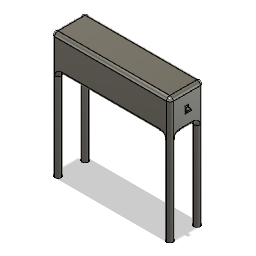
cat v1 (Autodesk Fusion 360 design; units mm, degrees)
Autodesk Fusion 360 part; units mm, degrees
sketch "Sketch1" plane through (0, 0, 0) normal (0, 1, 0) x (1, 0, 0)
  line L0 (0, 0) -> (350, 0)
  line L1 (350, 0) -> (350, 100)
  line L2 (350, 100) -> (0, 100)
  line L3 (0, 100) -> (0, 0)
  line L4 (0, 0) -> (20, 0)
  line L5 (20, 0) -> (20, 20)
  line L6 (20, 20) -> (0, 20)
  line L7 (0, 20) -> (0, 0)
  line L8 (0, 100) -> (20, 100)
  line L9 (20, 100) -> (20, 80)
  line L10 (20, 80) -> (0, 80)
  line L11 (0, 80) -> (0, 100)
  line L12 (350, 100) -> (330, 100)
  line L13 (330, 100) -> (330, 80)
  line L14 (330, 80) -> (350, 80)
  line L15 (350, 80) -> (350, 100)
  line L16 (350, 0) -> (330, 0)
  line L17 (330, 0) -> (330, 20)
  line L18 (330, 20) -> (350, 20)
  line L19 (350, 20) -> (350, 0)
  dimension "d1" = 350
  dimension "d2" = 100
  dimension "d3" = 20
  dimension "d4" = 20
  dimension "d5" = 20
  dimension "d6" = 20
  dimension "d7" = 20
  dimension "d8" = 20
  dimension "d9" = 20
  dimension "d10" = 20
  constraint horizontal L0
  constraint vertical L1
  constraint horizontal L2
  constraint vertical L3
  constraint coincident L0.start L3.end
  constraint horizontal L4
  constraint vertical L5
  constraint horizontal L6
  constraint vertical L7
  constraint horizontal L8
  constraint vertical L9
  constraint horizontal L10
  constraint vertical L11
  constraint horizontal L12
  constraint vertical L13
  constraint horizontal L14
  constraint vertical L15
  constraint horizontal L16
  constraint vertical L17
  constraint horizontal L18
  constraint vertical L19
  measures "d1" distance of L0.start L0.end
  measures "d2" distance of L0.start L2.end
  measures "d3" distance of L0.start L4.end
  measures "d4" distance of L0.start L6.end
  measures "d5" distance of L2.end L8.end
  measures "d6" distance of L2.end L10.end
  measures "d7" distance of L1.end L12.end
  measures "d8" distance of L1.end L14.end
  measures "d9" distance of L0.end L16.end
  measures "d10" distance of L0.end L18.end
extrude "Extrude1" add sketch "Sketch1" along normal blind 100 makes body 1
sketch "Sketch2" plane through (0, 0, 0) normal (0, -1, 0) x (1, 0, 0)
  line L0 (350, -100) -> (350, 0)
  line L1 (350, 0) -> (0, 0)
  line L2 (0, 0) -> (0, -100)
  line L3 (0, -100) -> (350, -100)
  line L4 (350, -100) -> (330, -100)
  line L5 (330, -100) -> (330, -80)
  line L6 (330, -80) -> (350, -80)
  line L7 (350, -80) -> (350, -100)
  line L8 (350, 0) -> (330, 0)
  line L9 (330, 0) -> (330, -20)
  line L10 (330, -20) -> (350, -20)
  line L11 (350, -20) -> (350, 0)
  line L12 (0, 0) -> (20, 0)
  line L13 (20, 0) -> (20, -20)
  line L14 (20, -20) -> (0, -20)
  line L15 (0, -20) -> (0, 0)
  line L16 (0, -100) -> (20, -100)
  line L17 (20, -100) -> (20, -80)
  line L18 (20, -80) -> (0, -80)
  line L19 (0, -80) -> (0, -100)
  dimension "d13" = 20
  dimension "d14" = 20
  dimension "d15" = 20
  dimension "d16" = 20
  dimension "d17" = 20
  dimension "d18" = 20
  dimension "d19" = 20
  dimension "d20" = 20
  constraint horizontal L4
  constraint vertical L5
  constraint horizontal L6
  constraint vertical L7
  constraint coincident L0.start L3.end
  constraint horizontal L8
  constraint vertical L9
  constraint horizontal L10
  constraint vertical L11
  constraint coincident L0.end L1.start
  constraint horizontal L12
  constraint vertical L13
  constraint horizontal L14
  constraint vertical L15
  constraint coincident L1.end L2.start
  constraint horizontal L16
  constraint vertical L17
  constraint horizontal L18
  constraint vertical L19
  constraint coincident L2.end L3.start
  measures "d13" distance of L0.start L4.end
  measures "d14" distance of L0.start L6.end
  measures "d15" distance of L0.end L8.end
  measures "d16" distance of L0.end L10.end
  measures "d17" distance of L1.end L12.end
  measures "d18" distance of L1.end L14.end
  measures "d19" distance of L2.end L16.end
  measures "d20" distance of L2.end L18.end
extrude "Extrude2" add sketch "Sketch2" along normal blind 300 contours L0 L3 L4 L5 L6 L7 | L0 L1 L8 L9 L10 L11 | L2 L3 L16 L17 L18 L19 | L1 L2 L12 L13 L14 L15 bodies 1
move_body "Move1" bodies 1 to x (1, 0, 0) y (0, 1, 0) z (0, 0, 1) at (0, 300, 0)
fillet "Fillet1" radius 9.9 40 edges at (350, 200, 0) (20, 150, 0) (20, 300, -10) (175, 300, 0) (330, 300, -90) (330, 0, -90) (340, 300, -80) (0, 0, -10) (0, 200, 0) (350, 400, -50) (350, 300, -50) (330, 0, -10) (330, 300, -10) (340, 300, -20) (350, 0, -90) (350, 0, -10) (330, 150, 0) (0, 150, -80) (350, 150, -20) (0, 300, -50) (350, 150, -80) (0, 150, -20) (175, 400, -100) (175, 400, 0) (330, 150, -100) (0, 200, -100) (330, 150, -20) (0, 400, -50) (330, 150, -80) (0, 0, -90) (350, 200, -100) (20, 150, -80) (20, 0, -90) (20, 0, -10) (20, 150, -20) (10, 300, -20) (10, 300, -80) (20, 300, -90) (175, 300, -100) (20, 150, -100) on bodies 1
sketch "Sketch3" plane through (0, 0, 0) normal (0, 1, 0) x (1, 0, 0)
  line L0 (-15, 5) -> (385, 5)
  line L1 (385, 5) -> (385, 15)
  line L2 (385, 15) -> (-15, 15)
  line L3 (-15, 15) -> (-15, 5)
  dimension "d25" = 400
  dimension "d26" = 10
  constraint horizontal L0
  constraint vertical L1
  constraint horizontal L2
  constraint vertical L3
  measures "d25" distance of L0.start L0.end
  measures "d26" distance of L0.start L2.end
extrude "Extrude3" cut sketch "Sketch3" along normal blind 30 bodies 1
sketch "Sketch4" plane through (0, 0, 0) normal (0, 1, 0) x (1, 0, 0)
  line L0 (-15, 95) -> (385, 95)
  line L1 (385, 95) -> (385, 85)
  line L2 (385, 85) -> (-15, 85)
  line L3 (-15, 85) -> (-15, 95)
  dimension "d29" = 400
  dimension "d30" = 10
  constraint horizontal L0
  constraint vertical L1
  constraint horizontal L2
  constraint vertical L3
  measures "d29" distance of L0.start L0.end
  measures "d30" distance of L0.start L2.end
extrude "Extrude4" cut sketch "Sketch4" along normal blind 30 bodies 1
sketch "Sketch5" plane through (0, 0, 0) normal (-1, 0, 0) x (0, 0, 1)
  line L0 (-90.1, 30) -> (-89.9, 30)
  line L1 (-89.9, 30) -> (-89.9, 290.1)
  arc A0 (-70.1, 309.9) -> (-89.9, 290.1) centre (-70.1, 290.1) ccw
  line L2 (-70.1, 309.9) -> (-29.9, 309.9)
  arc A1 (-10.1, 290.1) -> (-29.9, 309.9) centre (-29.9, 290.1) ccw
  line L3 (-10.1, 290.1) -> (-10.1, 30)
  line L4 (-10.1, 30) -> (-9.9, 30)
  line L5 (-9.9, 30) -> (-9.9, 390.1)
  line L6 (-9.9, 390.1) -> (-90.1, 390.1)
  line L7 (-90.1, 390.1) -> (-90.1, 30)
  circle A2 centre (-50, 350) radius 25
  line L8 (-70.1, 364.8657) -> (-85, 360)
  line L9 (-85, 360) -> (-75, 350)
  line L10 (-29.9, 364.8657) -> (-15, 360)
  line L11 (-15, 360) -> (-25, 350)
  line L12 (-45, 345) -> (-40, 350)
  line L13 (-40, 350) -> (-30, 350)
  line L14 (-30, 350) -> (-35, 345)
  line L15 (-35, 345) -> (-45, 345)
  line L16 (-55, 345) -> (-60, 350)
  line L17 (-60, 350) -> (-70, 350)
  line L18 (-70, 350) -> (-65, 345)
  line L19 (-65, 345) -> (-55, 345)
  line L20 (-48, 342) -> (-52, 342)
  line L21 (-52, 342) -> (-50, 340)
  line L22 (-50, 340) -> (-48, 342)
  line L23 (-50, 337) -> (-47, 335)
  line L24 (-47, 335) -> (-45, 336)
  line L25 (-45, 336) -> (-45, 335)
  line L26 (-45, 335) -> (-47, 334)
  line L27 (-47, 334) -> (-50, 336)
  line L28 (-50, 336) -> (-53, 334)
  line L29 (-53, 334) -> (-55, 335)
  line L30 (-55, 335) -> (-55, 336)
  line L31 (-55, 336) -> (-53, 335)
  line L32 (-53, 335) -> (-50, 337)
  dimension "d33" = 50
  constraint coincident A2 L8.start
  constraint coincident A2 L9.end
  constraint coincident A2 L10.start
  constraint coincident A2 L11.end
  constraint parallel L11 L12
  constraint horizontal L13
  constraint parallel L12 L14
  constraint parallel L13 L15
  constraint perpendicular L12 L16
  constraint parallel L15 L17
  constraint parallel L16 L18
  constraint parallel L17 L19
  constraint horizontal L20
  constraint perpendicular L21 L22
  constraint vertical L25
  constraint parallel L24 L26
  constraint vertical L30
  constraint parallel L29 L31
  measures "d33" diameter of A2
extrude "Extrude5" add sketch "Sketch5" along normal blind 5 contours A2 | A2 L10 L11 | A2 L8 L9 bodies 1
sketch "Sketch6" plane through (350, 0, 0) normal (1, 0, 0) x (0, 0, -1)
  line L0 (89.9, 30) -> (90.1, 30)
  line L1 (90.1, 30) -> (90.1, 390.1)
  line L2 (90.1, 390.1) -> (9.9, 390.1)
  line L3 (9.9, 390.1) -> (9.9, 30)
  line L4 (9.9, 30) -> (10.1, 30)
  line L5 (10.1, 30) -> (10.1, 290.1)
  arc A0 (29.9, 309.9) -> (10.1, 290.1) centre (29.9, 290.1) ccw
  line L6 (29.9, 309.9) -> (70.1, 309.9)
  arc A1 (89.9, 290.1) -> (70.1, 309.9) centre (70.1, 290.1) ccw
  line L7 (89.9, 290.1) -> (89.9, 30)
  line L8 (55, 360) -> (45, 360)
  line L9 (45, 360) -> (45, 340)
  line L10 (45, 340) -> (55, 340)
  line L11 (55, 340) -> (55, 360)
  constraint horizontal L8
  constraint vertical L9
  constraint horizontal L10
  constraint vertical L11
extrude "Extrude6" cut sketch "Sketch6" against normal blind 2 contours L8 L9 L10 L11 bodies 1
sketch "Sketch7" plane through (348, 0, 0) normal (1, 0, 0) x (0, 0, -1)
  line L0 (55, 340) -> (55, 360)
  line L1 (55, 360) -> (45, 360)
  line L2 (45, 360) -> (45, 340)
  line L3 (45, 340) -> (55, 340)
  line L4 (55, 352.0722) -> (45, 352.0722)
  line L5 (45, 352.0722) -> (45, 348.0722)
  line L6 (45, 348.0722) -> (55, 348.0722)
  line L7 (55, 348.0722) -> (55, 352.0722)
  dimension "d38" = 10
  dimension "d39" = 4
  constraint horizontal L4
  constraint vertical L5
  constraint horizontal L6
  constraint vertical L7
  constraint coincident L0 L4.start
  measures "d38" distance of L4.start L4.end
  measures "d39" distance of L4.start L6.end
extrude "Extrude7" add sketch "Sketch7" along normal blind 10 separate body contours L0 L2 L4 L5 L6 L7 makes body 2
extrude "Extrude8" cut 1 faces at (342.9008, 21.6667, -85) along direction (0, 0, -1) blind 45 on bodies 1 bodies 1
extrude "Extrude9" cut 1 faces at (12.9008, 21.6667, -5) along direction (0, 0, -1) blind 155 on bodies 1 bodies 1
extrude "Extrude10" cut 1 faces at (12.9008, 21.6667, -5) along direction (0, 0, 1) blind 50 on bodies 1 bodies 1
extrude "Extrude11" cut 1 faces at (342.9008, 21.6667, -85) along direction (0, 0, 1) blind 130 on bodies 1 bodies 1
